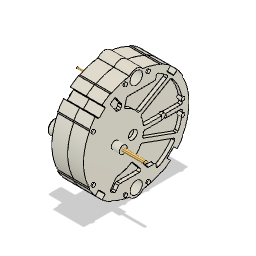
X27-168-Stepper v5 (Autodesk Fusion 360 design; units mm, degrees)
Autodesk Fusion 360 part; units mm, degrees
sketch "Sketch1" plane through (0, 0, 0) normal (1, 0, 0) x (0, 0, -1)
  line L0 (-4.4067, -0.8601) -> (-4.4067, 18.5277) construction
  line L1 (-4.4067, -0.8601) -> (-4.4067, -19.8773) construction
  line L2 (-4.4067, -0.8601) -> (21.636, -0.8601) construction
  line L3 (-4.4067, -0.8601) -> (-24.4318, -0.8601) construction
  arc A0 (-2.5017, 14.0184) -> (-6.3118, 14.0184) centre (-4.4067, 12.6425) ccw
  arc A1 (-6.3145, -15.7383) -> (-2.4989, -15.7383) centre (-4.4067, -14.3661) ccw
  line L4 (2.5631, 12.4223) -> (2.9837, 12.4223)
  line L5 (8.873, 6.5351) -> (8.873, 6.1148)
  line L6 (8.873, -7.835) -> (8.873, -8.2553)
  line L7 (2.9927, -14.1374) -> (2.5727, -14.1374)
  line L8 (-11.3861, -14.1374) -> (-11.8062, -14.1374)
  line L9 (-17.6759, -7.8551) -> (-17.6759, -8.2743)
  line L10 (-17.6759, 6.5541) -> (-17.6759, 6.1349)
  line L11 (-11.8062, 12.4172) -> (-11.3861, 12.4172)
  arc A2 (-6.3118, 14.0184) -> (-11.3861, 12.4172) centre (-4.4067, -0.8601) ccw
  arc A3 (-17.6759, 6.1349) -> (-17.6759, -7.8551) centre (-4.4067, -0.8601) ccw
  arc A4 (-11.3861, -14.1374) -> (-6.3145, -15.7383) centre (-4.4067, -0.8601) ccw
  arc A5 (-2.4989, -15.7383) -> (2.5727, -14.1374) centre (-4.4067, -0.8601) ccw
  arc A6 (8.873, -7.835) -> (8.873, 6.1148) centre (-4.4067, -0.8601) ccw
  arc A7 (2.5631, 12.4223) -> (-2.5017, 14.0184) centre (-4.4067, -0.8601) ccw
  circle A8 centre (-4.4067, 12.6425) radius 0.9209
  circle A9 centre (-4.4067, 12.6425) radius 1.2263
  circle A10 centre (-4.4067, 12.6425) radius 1.5619
  circle A11 centre (-4.4067, 12.6425) radius 1.7817
  circle A12 centre (-10.4097, -0.8601) radius 1
  circle A13 centre (-10.4097, -0.8601) radius 1.1043
  circle A14 centre (-10.4097, -0.8601) radius 0.9029
  circle A15 centre (-10.4097, -0.8601) radius 0.5
  circle A16 centre (-4.4067, -14.3661) radius 1.75
  circle A17 centre (-4.4067, -14.3661) radius 1.5597
  circle A18 centre (-4.4067, -14.3661) radius 1.2196
  circle A19 centre (-4.4067, -14.3661) radius 0.9326
  circle A20 centre (-7.6531, -14.4857) radius 0.5
  circle A21 centre (-1.16, -14.4857) radius 0.5
  circle A22 centre (-1.1623, 12.7607) radius 0.5
  circle A23 centre (-7.6764, 12.7607) radius 0.5
  circle A24 centre (8.641, 1.1394) radius 0.5
  circle A25 centre (8.6402, -2.8729) radius 0.5
  circle A26 centre (-16.7858, -7.4196) radius 0.5
  circle A27 centre (-16.789, 5.6908) radius 0.5
  circle A28 centre (-5.3601, -0.8601) radius 1.25
  circle A29 centre (3.4058, -0.8601) radius 0.75
  line L12 (2.8964, -0.3096) -> (-1.9645, -0.3096)
  line L13 (-2.8122, 2.8822) -> (5.233, 7.5224)
  line L14 (3.9018, -0.2975) -> (8.2503, -0.2975)
  line L15 (8.6971, 0.1445) -> (8.6743, 0.6405)
  arc A30 (8.2503, -0.2975) -> (8.6971, 0.1445) centre (8.2742, 0.1251) ccw
  arc A31 (-2.4073, 0.0969) -> (-1.9645, -0.3096) centre (-1.9645, 0.1348) ccw
  arc A32 (-2.4073, 0.0969) -> (-3.0084, 2.3264) centre (-8.9083, -0.46) ccw
  arc A33 (-2.8122, 2.8822) -> (-3.0084, 2.3264) centre (-2.5858, 2.4897) ccw
  arc A34 (5.7979, 7.4181) -> (5.233, 7.5224) centre (5.4542, 7.1389) ccw
  arc A35 (8.5331, 1.6276) -> (5.7979, 7.4181) centre (-4.6199, -1.0441) ccw
  line L16 (2.9074, -1.4205) -> (-1.9603, -1.4205)
  arc A36 (-1.9603, -1.4205) -> (-2.4022, -1.8018) centre (-1.9603, -1.8673) ccw
  arc A37 (-2.5612, -2.705) -> (-2.4022, -1.8018) centre (-5.829, -1.6642) ccw
  arc A38 (-2.5612, -2.705) -> (-2.2776, -3.228) centre (-2.1681, -2.8302) ccw
  line L17 (-2.2776, -3.228) -> (6.9763, -6.5951)
  arc A39 (6.9763, -6.5951) -> (7.5084, -6.3904) centre (7.1248, -6.1871) ccw
  arc A40 (7.5084, -6.3904) -> (8.5209, -3.3585) centre (-1.0924, -1.8332) ccw
  line L18 (-2.657, -4.2788) -> (6.2953, -7.5343)
  line L19 (-4.5555, -6.9779) -> (-1.2541, -10.8992)
  line L20 (-0.9101, -11.0649) -> (0.6697, -11.0649)
  arc A41 (-2.657, -4.2788) -> (-3.2095, -4.4917) centre (-2.8111, -4.7025) ccw
  arc A42 (-4.5302, -6.3861) -> (-3.2095, -4.4917) centre (-11.5739, -0.0679) ccw
  arc A43 (-4.5302, -6.3861) -> (-4.5555, -6.9779) centre (-4.2204, -6.6958) ccw
  arc A44 (-1.2541, -10.8992) -> (-0.9101, -11.0649) centre (-0.9101, -10.6248) ccw
  arc A45 (1.2294, -11.6221) -> (0.6697, -11.0649) centre (0.6697, -11.6246) ccw
  arc A46 (1.2294, -11.6221) -> (1.24, -12.0198) centre (10.2849, -11.5808) ccw
  arc A47 (1.24, -12.0198) -> (1.888, -12.4055) centre (1.6687, -12.0367) ccw
  arc A48 (1.888, -12.4055) -> (6.5021, -8.2019) centre (-4.3755, -0.8963) ccw
  arc A49 (6.5021, -8.2019) -> (6.2953, -7.5343) centre (6.1453, -7.9466) ccw
  line L21 (3.9081, -1.417) -> (8.2552, -1.417)
  line L22 (8.6952, -1.8597) -> (8.671, -2.3738)
  arc A50 (8.6952, -1.8597) -> (8.2552, -1.417) centre (8.2552, -1.857) ccw
  arc A51 (-9.8026, -8.9004) -> (-5.9889, -7.6178) centre (-10.4198, -0.7543) ccw
  arc A52 (-5.4059, -7.6932) -> (-5.9889, -7.6178) centre (-5.742, -8.0002) ccw
  arc A53 (-3.1904, -10.3408) -> (-5.4059, -7.6932) centre (-34.8025, -34.5427) ccw
  arc A54 (-3.5059, -11.0679) -> (-3.1904, -10.3408) centre (-3.5126, -10.633) ccw
  arc A55 (-8.9589, -11.0679) -> (-3.5059, -11.0679) centre (-6.2324, 166.0207) ccw
  arc A56 (-8.9589, -11.0679) -> (-9.4459, -11.3011) centre (-8.9682, -11.6735) ccw
  arc A57 (-9.4459, -11.3011) -> (-10.1249, -12.2545) centre (1.2154, -19.6129) ccw
  arc A58 (-10.7148, -12.4054) -> (-10.1249, -12.2545) centre (-10.5017, -12.01) ccw
  arc A59 (-11.5242, -11.9253) -> (-10.7148, -12.4054) centre (-5.2803, -2.3221) ccw
  arc A60 (-11.6751, -11.2874) -> (-11.5242, -11.9253) centre (-11.2794, -11.5306) ccw
  arc A61 (-10.1318, -9.0993) -> (-11.6751, -11.2874) centre (6.3834, -22.3862) ccw
  arc A62 (-9.8026, -8.9004) -> (-10.1318, -9.0993) centre (-9.7703, -9.3257) ccw
  line L23 (-16.0708, 8.8862) -> (-15.1488, 7.9637)
  line L24 (-14.9498, 8.0007) -> (-13.2614, 9.6883)
  line L25 (-13.274, 9.873) -> (-14.1646, 10.7942)
  arc A63 (-13.2614, 9.6883) -> (-13.274, 9.873) centre (-13.3772, 9.7732) ccw
  arc A64 (-15.1488, 7.9637) -> (-14.9498, 8.0007) centre (-15.0762, 8.1271) ccw
  arc A65 (-11.8062, 12.4172) -> (-14.1646, 10.7942) centre (-4.4067, -0.8601) ccw
  arc A66 (-16.0708, 8.8862) -> (-17.6759, 6.5541) centre (-4.4067, -0.8601) ccw
  arc A67 (5.3368, 10.8063) -> (4.4145, 9.8899) centre (27.3451, -12.2651) ccw
  arc A68 (4.4145, 9.8899) -> (4.4326, 9.7023) centre (4.4478, 9.7984) ccw
  arc A69 (6.1572, 7.9777) -> (4.4326, 9.7023) centre (-158.4507, -154.9056) ccw
  arc A70 (6.1572, 7.9777) -> (6.3071, 7.9895) centre (6.2246, 8.0786) ccw
  arc A71 (6.3071, 7.9895) -> (7.2502, 8.8947) centre (-0.3735, 15.8934) ccw
  arc A72 (8.873, 6.5351) -> (7.2502, 8.8947) centre (-4.4067, -0.8601) ccw
  arc A73 (5.3368, 10.8063) -> (2.9837, 12.4223) centre (-4.4067, -0.8601) ccw
  arc A74 (4.4051, -11.6064) -> (5.3401, -12.5237) centre (93.0217, 77.7849) ccw
  arc A75 (4.4513, -11.4172) -> (4.4051, -11.6064) centre (4.5901, -11.5514) ccw
  arc A76 (6.1786, -9.7208) -> (4.4513, -11.4172) centre (37.8756, -43.7201) ccw
  arc A77 (6.3203, -9.7271) -> (6.1786, -9.7208) centre (6.2457, -9.8075) ccw
  arc A78 (7.2537, -10.6107) -> (6.3203, -9.7271) centre (-39.755, -59.3372) ccw
  arc A79 (2.9927, -14.1374) -> (5.3401, -12.5237) centre (-4.4067, -0.8601) ccw
  arc A80 (7.2537, -10.6107) -> (8.873, -8.2553) centre (-4.4067, -0.8601) ccw
  arc A81 (-15.1488, -9.7243) -> (-16.0692, -10.6082) centre (-5.0124, -21.2003) ccw
  arc A82 (-14.9454, -9.7291) -> (-15.1488, -9.7243) centre (-15.0489, -9.8031) ccw
  arc A83 (-13.2817, -11.4119) -> (-14.9454, -9.7291) centre (-46.5076, -42.5964) ccw
  arc A84 (-13.2578, -11.584) -> (-13.2817, -11.4119) centre (-13.4029, -11.5164) ccw
  arc A85 (-14.1561, -12.5216) -> (-13.2578, -11.584) centre (-20.4506, -5.5922) ccw
  arc A86 (-17.6759, -8.2743) -> (-16.0692, -10.6082) centre (-4.4067, -0.8601) ccw
  arc A87 (-14.1561, -12.5216) -> (-11.8062, -14.1374) centre (-4.4067, -0.8601) ccw
  arc A88 (-10.1272, 10.5419) -> (-10.7174, 10.6683) centre (-10.4863, 10.3064) ccw
  arc A89 (-10.1272, 10.5419) -> (-8.6611, 8.4443) centre (26.1036, 34.3038) ccw
  arc A90 (-8.595, 8.0705) -> (-8.6611, 8.4443) centre (-9.0012, 8.1914) ccw
  arc A91 (-8.7618, 7.4428) -> (-8.595, 8.0705) centre (-11.0051, 8.375) ccw
  arc A92 (-9.2418, 7.1203) -> (-8.7618, 7.4428) centre (-9.1833, 7.5518) ccw
  arc A93 (-9.2418, 7.1203) -> (-9.7843, 7.1659) centre (-9.9605, 1.8107) ccw
  arc A94 (-10.0983, 7.3542) -> (-9.7843, 7.1659) centre (-9.7719, 7.5424) ccw
  arc A95 (-11.6504, 9.5631) -> (-10.0983, 7.3542) centre (51.3201, 52.1619) ccw
  arc A96 (-11.5125, 10.2016) -> (-11.6504, 9.5631) centre (-11.2752, 9.8162) ccw
  arc A97 (-11.5125, 10.2016) -> (-10.7174, 10.6683) centre (-17.3665, 21.0846) ccw
  line L26 (-6.7552, 9.3329) -> (0.6688, 9.3329)
  line L27 (-3.3795, 3.8493) -> (4.2578, 8.2578)
  line L28 (-7.1916, 9.0071) -> (-7.6798, 7.1524)
  arc A98 (-6.7552, 9.3329) -> (-7.1916, 9.0071) centre (-6.7552, 8.8777) ccw
  arc A99 (-7.6798, 7.1524) -> (-7.4357, 6.6248) centre (-7.2386, 7.0363) ccw
  arc A100 (-3.9549, 3.958) -> (-7.4357, 6.6248) centre (-10.2458, -0.6481) ccw
  arc A101 (-3.9549, 3.958) -> (-3.3795, 3.8493) centre (-3.604, 4.2383) ccw
  arc A102 (4.2578, 8.2578) -> (4.3323, 8.9474) centre (4.0431, 8.6298) ccw
  arc A103 (4.3323, 8.9474) -> (1.889, 10.6745) centre (-3.8525, -0.0399) ccw
  arc A104 (1.889, 10.6745) -> (1.2328, 10.2865) centre (1.6761, 10.2856) ccw
  arc A105 (1.2304, 9.8864) -> (1.2328, 10.2865) centre (-48.5104, 10.3841) ccw
  arc A106 (0.6688, 9.3329) -> (1.2304, 9.8864) centre (0.6688, 9.8946) ccw
  dimension "d1" = 30
  dimension "d2" = 4.7
  dimension "d3" = 4.7
  dimension "d4" = 30.4
  dimension "d5" = 2
  dimension "d6" = 1
  dimension "d7" = 3.5
  dimension "d8" = 1
  dimension "d9" = 1
  dimension "d10" = 1
  dimension "d11" = 1
  dimension "d12" = 1
  dimension "d13" = 1
  dimension "d14" = 1
  dimension "d15" = 1
  dimension "d16" = 2.5
  dimension "d17" = 1.5
  constraint coincident L0.start L1.start
  constraint vertical L0
  constraint parallel L0 L1
  constraint perpendicular L0 L2
  constraint perpendicular L1 L3
  constraint coincident L0 A0.centre
  constraint coincident L1 A1.centre
  constraint coincident A1.end A2
  constraint concentric A2 A5
  constraint concentric A5 A65
  constraint coincident L4.start A5
  constraint horizontal L4
  constraint coincident L5.start A65
  constraint coincident L5.end A5
  constraint vertical L5
  constraint coincident L6.start A5
  constraint coincident L6.end A65
  constraint parallel L5 L6
  constraint coincident L7.start A65
  constraint perpendicular L5 L7
  constraint coincident L8.start A2
  constraint coincident L8.end A65
  constraint parallel L7 L8
  constraint coincident L9.start A2
  constraint coincident L9.end A65
  constraint perpendicular L8 L9
  constraint coincident L10.end A2
  constraint perpendicular L8 L10
  constraint perpendicular L10 L11
  constraint concentric A2 A3
  constraint concentric A65 A86
  constraint concentric A3 A4
  constraint concentric A79 A86
  constraint concentric A5 A6
  constraint concentric A72 A79
  constraint concentric A6 A7
  constraint concentric A0 A8
  constraint concentric A8 A9
  constraint concentric A8 A10
  constraint concentric A0 A11
  constraint coincident L3 A12.centre
  constraint concentric A12 A13
  constraint concentric A13 A14
  constraint concentric A14 A15
  constraint concentric A1 A16
  constraint concentric A16 A17
  constraint concentric A1 A18
  constraint concentric A16 A19
  constraint coincident L3 A28.centre
  constraint coincident L2 A29.centre
  constraint coincident A29 L12.start
  constraint horizontal L12
  constraint coincident A29 L14.start
  constraint horizontal L14
  constraint coincident A24 L15.end
  constraint tangent L15 A30
  constraint tangent L12 A31
  constraint tangent A31 A32
  constraint tangent L13 A33
  constraint tangent L13 A34
  constraint tangent A34 A35
  constraint coincident A24 A35.start
  constraint coincident A29 L16.start
  constraint parallel L12 L16
  constraint tangent L16 A36
  constraint tangent A37 A38
  constraint tangent L17 A39
  constraint tangent A39 A40
  constraint coincident A25 A40.end
  constraint horizontal L20
  constraint tangent L18 A41
  constraint tangent A41 A42
  constraint tangent L19 A43
  constraint tangent L20 A44
  constraint tangent L20 A45
  constraint tangent A45 A46
  constraint tangent L18 A49
  constraint coincident A29 L21.start
  constraint parallel L2 L21
  constraint coincident A25 L22.end
  constraint tangent L21 A50
  constraint tangent A51 A52
  constraint tangent A52 A53
  constraint tangent A54 A55
  constraint tangent A55 A56
  constraint tangent A56 A57
  constraint tangent A57 A58
  constraint tangent A58 A59
  constraint tangent A58 A60
  constraint tangent A60 A61
  constraint tangent A51 A62
  constraint coincident L23.start A65
  constraint perpendicular L23 L24
  constraint tangent L25 A63
  constraint tangent L24 A64
  constraint concentric A65 A66
  constraint coincident A67.start A72
  constraint concentric A72 A73
  constraint tangent A75 A76
  constraint tangent A77 A78
  constraint coincident A78.start A79
  constraint concentric A79 A80
  constraint coincident A85.start A86
  constraint concentric A86 A87
  constraint tangent A88 A89
  constraint tangent A89 A90
  constraint tangent A88 A91
  constraint tangent A92 A93
  constraint tangent A93 A94
  constraint tangent A88 A97
  constraint horizontal L26
  constraint tangent L26 A98
  constraint tangent L28 A99
  constraint tangent L27 A101
  constraint tangent L27 A102
  constraint tangent A102 A103
  constraint tangent A104 A105
  constraint tangent L26 A106
  measures "d1" diameter of A2
  measures "d2" diameter of A0
  measures "d3" diameter of A1
  measures "d4" diameter of A65
  measures "d5" diameter of A12
  measures "d6" diameter of A15
  measures "d7" diameter of A16
  measures "d8" diameter of A20
  measures "d9" diameter of A21
  measures "d10" diameter of A22
  measures "d11" diameter of A23
  measures "d12" diameter of A24
  measures "d13" diameter of A25
  measures "d14" diameter of A26
  measures "d15" diameter of A27
  measures "d16" diameter of A28
  measures "d17" diameter of A29
extrude "Extrude1" add sketch "Sketch1" against normal blind 9 contours A0 A1 L4 L5 L6 L7 L8 L9 L10 L11 A2 A3 A4 A5 A6 A7 L23 L24 L25 A63 A64 A65 A66 A67 A68 A69 A70 A71 A72 A73 A74 A75 A76 A77 A78 A79 A80 A81 A82 A83 A84 A85 A86 A87 | A8 | A9 | A10 | A11 | A12 | A13 | A14 | A15 | A16 | A17 | A18 | A19 | A20 | A21 | A22 | A23 | A24 | A24 A29 L12 L13 L14 L15 A30 A31 A32 A33 A34 A35 | A29 | A25 A29 L16 A36 A37 A38 L17 A39 A40 L21 L22 A50 | A25 | A26 | A27 | A28 | L18 L19 L20 A41 A42 A43 A44 A45 A46 A47 A48 A49 | A51 A52 A53 A54 A55 A56 A57 A58 A59 A60 A61 A62 | A88 A89 A90 A91 A92 A93 A94 A95 A96 A97 | L26 L27 L28 A98 A99 A100 A101 A102 A103 A104 A105 A106 makes body 1
extrude "Extrude2" cut sketch "Sketch1" against normal blind 1 contours A24 A29 L12 L13 L14 L15 A30 A31 A32 A33 A34 A35 | A25 A29 L16 A36 A37 A38 L17 A39 A40 L21 L22 A50 | L18 L19 L20 A41 A42 A43 A44 A45 A46 A47 A48 A49 | A51 A52 A53 A54 A55 A56 A57 A58 A59 A60 A61 A62 | A88 A89 A90 A91 A92 A93 A94 A95 A96 A97 | L26 L27 L28 A98 A99 A100 A101 A102 A103 A104 A105 A106 bodies 1
extrude "Extrude3" cut sketch "Sketch1" against normal blind 4.5 contours A8 | A9 | A10 | A11 bodies 1
extrude "Extrude4" cut sketch "Sketch1" against normal blind 10 contours A8 bodies 1
extrude "Extrude5" cut sketch "Sketch1" against normal blind 4.5 contours A16 | A17 | A18 | A19 bodies 1
extrude "Extrude6" cut sketch "Sketch1" against normal blind 10 contours A19 bodies 1
extrude "Extrude7" add sketch "Sketch1" along normal blind 0.3 contours A20 | A21 | A22 | A23 | A24 | A25 | A26 | A27 bodies 1
extrude "Extrude8" cut sketch "Sketch1" against normal blind 0.3 contours A29 bodies 1
extrude "Extrude9" cut sketch "Sketch1" against normal blind 1 contours A28 bodies 1
extrude "Extrude10" add sketch "Sketch1" along normal blind 2.3 contours A12 | A13 | A14 | A15 bodies 1
extrude "Extrude11" add sketch "Sketch1" along normal blind 9 separate body contours A15 makes body 2
chamfer "Chamfer1" distance 0.4 angle 45 1 edges at (9, -1.0409, 10.8759) on bodies 2
sketch "Sketch2" plane through (-9, 0, 0) normal (-1, 0, 0) x (0, 0, 1)
  circle A0 centre (4.4067, -14.3661) radius 0.9326
  circle A1 centre (4.4067, 12.6425) radius 0.9209
  arc A2 (13.2578, -11.584) -> (14.1561, -12.5216) centre (20.4506, -5.5922) ccw
  arc A3 (13.2817, -11.4119) -> (13.2578, -11.584) centre (13.4029, -11.5164) ccw
  arc A4 (14.9454, -9.7291) -> (13.2817, -11.4119) centre (46.5076, -42.5964) ccw
  arc A5 (15.1488, -9.7243) -> (14.9454, -9.7291) centre (15.0489, -9.8031) ccw
  arc A6 (16.0692, -10.6082) -> (15.1488, -9.7243) centre (5.0124, -21.2003) ccw
  arc A7 (16.0692, -10.6082) -> (17.6759, -8.2743) centre (4.4067, -0.8601) ccw
  line L0 (17.6759, -8.2743) -> (17.6759, -7.8551)
  arc A8 (17.6759, -7.8551) -> (17.6759, 6.1349) centre (4.4067, -0.8601) ccw
  line L1 (17.6759, 6.1349) -> (17.6759, 6.5541)
  arc A9 (17.6759, 6.5541) -> (16.0708, 8.8862) centre (4.4067, -0.8601) ccw
  line L2 (16.0708, 8.8862) -> (15.1488, 7.9637)
  arc A10 (14.9498, 8.0007) -> (15.1488, 7.9637) centre (15.0762, 8.1271) ccw
  line L3 (14.9498, 8.0007) -> (13.2614, 9.6883)
  arc A11 (13.274, 9.873) -> (13.2614, 9.6883) centre (13.3772, 9.7732) ccw
  line L4 (13.274, 9.873) -> (14.1646, 10.7942)
  arc A12 (14.1646, 10.7942) -> (11.8062, 12.4172) centre (4.4067, -0.8601) ccw
  line L5 (11.8062, 12.4172) -> (11.3861, 12.4172)
  arc A13 (11.3861, 12.4172) -> (6.3118, 14.0184) centre (4.4067, -0.8601) ccw
  arc A14 (6.3118, 14.0184) -> (2.5017, 14.0184) centre (4.4067, 12.6425) ccw
  arc A15 (2.5017, 14.0184) -> (-2.5631, 12.4223) centre (4.4067, -0.8601) ccw
  line L6 (-2.5631, 12.4223) -> (-2.9837, 12.4223)
  arc A16 (-2.9837, 12.4223) -> (-5.3368, 10.8063) centre (4.4067, -0.8601) ccw
  arc A17 (-4.4145, 9.8899) -> (-5.3368, 10.8063) centre (-27.3451, -12.2651) ccw
  arc A18 (-4.4326, 9.7023) -> (-4.4145, 9.8899) centre (-4.4478, 9.7984) ccw
  arc A19 (-4.4326, 9.7023) -> (-6.1572, 7.9777) centre (158.4507, -154.9056) ccw
  arc A20 (-6.3071, 7.9895) -> (-6.1572, 7.9777) centre (-6.2246, 8.0786) ccw
  arc A21 (-7.2502, 8.8947) -> (-6.3071, 7.9895) centre (0.3735, 15.8934) ccw
  arc A22 (-7.2502, 8.8947) -> (-8.873, 6.5351) centre (4.4067, -0.8601) ccw
  line L7 (-8.873, 6.5351) -> (-8.873, 6.1148)
  arc A23 (-8.873, 6.1148) -> (-8.873, -7.835) centre (4.4067, -0.8601) ccw
  line L8 (-8.873, -7.835) -> (-8.873, -8.2553)
  arc A24 (-8.873, -8.2553) -> (-7.2537, -10.6107) centre (4.4067, -0.8601) ccw
  arc A25 (-6.3203, -9.7271) -> (-7.2537, -10.6107) centre (39.755, -59.3372) ccw
  arc A26 (-6.1786, -9.7208) -> (-6.3203, -9.7271) centre (-6.2457, -9.8075) ccw
  arc A27 (-4.4513, -11.4172) -> (-6.1786, -9.7208) centre (-37.8756, -43.7201) ccw
  arc A28 (-4.4051, -11.6064) -> (-4.4513, -11.4172) centre (-4.5901, -11.5514) ccw
  arc A29 (-5.3401, -12.5237) -> (-4.4051, -11.6064) centre (-93.0217, 77.7849) ccw
  arc A30 (-5.3401, -12.5237) -> (-2.9927, -14.1374) centre (4.4067, -0.8601) ccw
  line L9 (-2.9927, -14.1374) -> (-2.5727, -14.1374)
  arc A31 (-2.5727, -14.1374) -> (2.4989, -15.7383) centre (4.4067, -0.8601) ccw
  arc A32 (2.4989, -15.7383) -> (6.3145, -15.7383) centre (4.4067, -14.3661) ccw
  arc A33 (6.3145, -15.7383) -> (11.3861, -14.1374) centre (4.4067, -0.8601) ccw
  line L10 (11.3861, -14.1374) -> (11.8062, -14.1374)
  arc A34 (11.8062, -14.1374) -> (14.1561, -12.5216) centre (4.4067, -0.8601) ccw
  arc A35 (-1.0377, -7.1782) -> (-1.0345, 5.4058) centre (-26.4034, -0.8798) ccw
  arc A36 (-0.0026, 6.5678) -> (-1.0345, 5.4058) centre (-0.1196, 5.6325) ccw
  arc A37 (-0.0026, 6.5678) -> (8.8766, 6.5711) centre (4.422, 47.5969) ccw
  arc A38 (9.8912, 5.4058) -> (8.8766, 6.5711) centre (8.9782, 5.6352) ccw
  arc A39 (9.8912, 5.4058) -> (9.8883, -7.1704) centre (34.9402, -0.888) ccw
  arc A40 (8.8766, -8.3434) -> (9.8883, -7.1704) centre (8.9696, -7.4008) ccw
  arc A41 (8.8766, -8.3434) -> (-0.0175, -8.3456) centre (4.4407, -53.3263) ccw
  arc A42 (-1.0377, -7.1782) -> (-0.0175, -8.3456) centre (-0.1204, -7.406) ccw
  arc A43 (-2.997, -8.248) -> (-3.0078, 6.467) centre (-26.528, -0.9077) ccw
  arc A44 (-3.0078, 6.467) -> (-3.7182, 7.1221) centre (-3.9071, 6.2045) ccw
  arc A45 (-4.7329, 7.3415) -> (-3.7182, 7.1221) centre (6.7761, 58.1143) ccw
  arc A46 (-4.4077, 8.9046) -> (-4.7329, 7.3415) centre (-4.5799, 8.1251) ccw
  arc A47 (-4.4077, 8.9046) -> (12.6671, 8.762) centre (4.4829, 51.1212) ccw
  arc A48 (12.5964, 7.1261) -> (13.0119, 7.2031) centre (4.7913, 50.3763) ccw
  arc A49 (12.5964, 7.1261) -> (11.8575, 6.4115) centre (12.7605, 6.2172) ccw
  arc A50 (11.8575, 6.4115) -> (11.8459, -8.2474) centre (34.8824, -0.9362) ccw
  arc A51 (11.8459, -8.2474) -> (12.5964, -8.8861) centre (12.7102, -7.9921) ccw
  arc A52 (13.6034, -9.1093) -> (12.5964, -8.8861) centre (11.8848, -14.4786) ccw
  arc A53 (13.2657, -10.6663) -> (13.6034, -9.1093) centre (13.4359, -9.8881) ccw
  arc A54 (13.2657, -10.6663) -> (-4.387, -10.6697) centre (4.447, -50.9752) ccw
  arc A55 (-4.723, -9.1073) -> (-4.387, -10.6697) centre (-4.5581, -9.8892) ccw
  arc A56 (-3.7296, -8.893) -> (-4.723, -9.1073) centre (-3.467, -12.5196) ccw
  arc A57 (-3.7296, -8.893) -> (-2.997, -8.248) centre (-3.7878, -8.0884) ccw
  circle A58 centre (13.4276, 8.1127) radius 1
  circle A59 centre (13.4276, 8.1127) radius 0.6875
  circle A60 centre (4.4067, 12.6425) radius 2.25
  circle A61 centre (4.4067, -14.3661) radius 2.25
  circle A62 centre (4.4067, -14.3661) radius 1.25
  circle A63 centre (4.4067, 12.6425) radius 1.25
  circle A64 centre (0.6086, 10.5315) radius 1.5
  circle A65 centre (0.6086, 10.5315) radius 0.9
  circle A66 centre (8.2306, 10.5315) radius 1.5
  circle A67 centre (8.2306, 10.5315) radius 0.9
  circle A68 centre (0.6086, -12.3285) radius 1.5
  circle A69 centre (0.6086, -12.3285) radius 0.9
  circle A70 centre (8.2306, -12.3285) radius 1.5
  circle A71 centre (8.2306, -12.3285) radius 0.9
  circle A72 centre (-8.0934, -5.8938) radius 0.75
  circle A73 centre (16.9066, -5.8938) radius 0.75
  circle A74 centre (-8.0934, 4.1062) radius 0.75
  circle A75 centre (16.9066, 4.1062) radius 0.75
  circle A76 centre (-8.0934, -5.8938) radius 0.25
  circle A77 centre (16.9066, -5.8938) radius 0.25
  circle A78 centre (-8.0934, 4.1062) radius 0.25
  circle A79 centre (16.9066, 4.1062) radius 0.25
  circle A80 centre (-5.5763, -0.8796) radius 2
  circle A81 centre (-5.5763, -0.8796) radius 1.5
  circle A82 centre (0.6086, 10.5315) radius 0.25
  circle A83 centre (8.2286, 10.5315) radius 0.25
  circle A84 centre (0.6086, -12.3285) radius 0.25
  circle A85 centre (8.2286, -12.3285) radius 0.25
  dimension "d41" = 2
  dimension "d42" = 1.375
  dimension "d47" = 4.5
  dimension "d48" = 4.5
  dimension "d49" = 2.5
  dimension "d50" = 2.5
  dimension "d51" = 3
  dimension "d52" = 1.8
  dimension "d55" = 7.622
  dimension "d56" = -22.86
  dimension "d57" = 1.5
  dimension "d60" = 25
  dimension "d61" = 10
  dimension "d62" = 0.5
  dimension "d65" = 25
  dimension "d66" = 10
  dimension "d67" = 4
  dimension "d68" = 3
  dimension "d73" = 0.5
  dimension "d76" = 7.62
  dimension "d77" = -22.86
  constraint tangent A35 A36
  constraint tangent A37 A38
  constraint tangent A38 A39
  constraint tangent A39 A40
  constraint tangent A40 A41
  constraint tangent A35 A42
  constraint tangent A44 A45
  constraint tangent A47 A48
  constraint tangent A48 A49
  constraint tangent A51 A52
  constraint tangent A53 A54
  constraint tangent A54 A55
  constraint tangent A56 A57
  constraint concentric A58 A59
  constraint coincident A58 A48.end
  constraint coincident A58 A47.end
  constraint concentric A1 A60
  constraint concentric A0 A61
  constraint concentric A61 A62
  constraint concentric A60 A63
  constraint concentric A64 A65
  constraint concentric A72 A76
  constraint concentric A80 A81
  constraint concentric A65 A82
  measures "d41" diameter of A58
  measures "d42" diameter of A59
  measures "d47" diameter of A60
  measures "d48" diameter of A61
  measures "d49" diameter of A62
  measures "d50" diameter of A63
  measures "d51" diameter of A64
  measures "d52" diameter of A65
  measures "d57" diameter of A72
  measures "d62" diameter of A76
  measures "d67" diameter of A80
  measures "d68" diameter of A81
  measures "d73" diameter of A82
extrude "Extrude12" add sketch "Sketch2" along normal blind 0.3 contours A43 A44 A45 A46 A47 A48 A49 A50 A51 A52 A53 A54 A55 A56 A57 A58 bodies 1
extrude "Extrude13" add sketch "Sketch2" along normal blind 4.7 contours L3 A58 | A59 picked at (14.0654, 8.7386) bodies 1
extrude "Extrude14" add sketch "Sketch2" along normal blind 4.4 contours A80 bodies 1
extrude "Extrude15" add sketch "Sketch2" along normal blind 0.3 contours A72 | A73 | A74 | A75 bodies 1
extrude "Extrude16" add sketch "Sketch2" along normal blind 0.3 contours A64 | A66 | A68 | A70 bodies 1
extrude "Extrude17" add sketch "Sketch2" along normal blind 4 separate body contours A82 | A83 | A84 | A85 makes body 3 at (-11.6667, -12.2313, 0.839) makes body 4 at (-11.6667, 10.6287, 0.839) makes body 5 at (-11.6667, -12.2429, 7.9937) makes body 6 at (-11.6667, 10.6171, 7.9937)
fillet "Fillet1" radius 0.3 1 edges at (-13.7, 7.4054, 12.7206) on bodies 1
chamfer "Chamfer2" distance 0.4 angle 45 1 edges at (-13.4, -1.6029, -7.441) on bodies 1
sketch "Sketch3" plane through (0, 0, 0) normal (1, 0, 0) x (0, 0, -1)
  line L0 (16.7624, 19.8845) -> (-29.7964, 19.8845)
  line L1 (-29.7964, 19.8845) -> (-29.7964, -21.2182)
  line L2 (-29.7964, -21.2182) -> (16.7624, -21.2182)
  line L3 (16.7624, -21.2182) -> (16.7624, 19.8845)
  constraint horizontal L0
  constraint vertical L1
  constraint horizontal L2
  constraint vertical L3
extrude "Extrude18" add sketch "Sketch3" against normal blind 0.01 separate body makes body 7
move_body "Move1" bodies 7 to x (1, 0, 0) y (0, 1, 0) z (0, 0, 1) at (-4.4861, 0, 0)
split "Split1" by plane through (-4.4861, 0, 0) normal (1, 0, 0) bodies 1 2 3 4 5 6 makes body 8 at (0, 4.3094, 12.3766)
move_body "Move2" bodies 1 3 4 5 6 to x (1, 0, 0) y (0, -1, 0) z (0, 0, -1) at (0, -1.733, 8.8135)
hidden bodies 7
named bodies: "Body_Top", "Needle", "Body_Top (1)"
